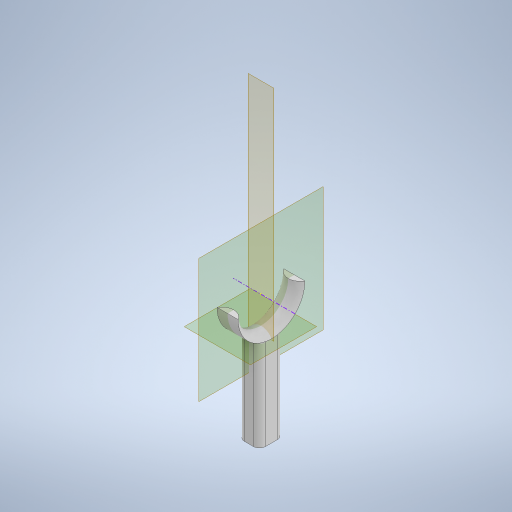
# Autodesk Inventor part: 막대1
Saved by Autodesk Inventor 2023 (Build 270158000, 158)
## iProperties
Created: 2023-04-26
Part Number: 막대1
Material: 일반
Document SubType Name: Modeling
Designer: rlatk
Density: 1 g/cm^3
Appearance: 기본값
Author: rlatk
Autodesk Inventor part; units mm, degrees
ref_plane "YZ Plane" through (0, 0, 0) normal (1, 0, 0) x (0, 1, 0)
ref_plane "XZ Plane" through (0, 0, 0) normal (0, 1, 0) x (-1, 0, 0)
sketch "스케치1" plane through (0, 0, 0) normal (0, 1, 0) x (-1, 0, 0)
  line L0 (0, 0) -> (3.5, 0)
  line L1 (0, 0) -> (-3.5, 0)
  arc A0 (3.5, 0) -> (-3.5, 0) centre (0, -1.9365) ccw
  line L2 (3.5, 0) -> (-3.5, 0)
  dimension "d1" = 3.5
  dimension "d2" = 4
  constraints: 6 end point, 2 point on circle, 1 centre point, 1 collinear, 1 horizontal
  measures "d1" distance of L0.start L0.end
  measures "d2" radius of A0
ref_plane "작업 평면4" through (0, 0, 11.1) normal (0, 0, 1) x (1, 0, 0)
sketch "스케치8" plane through (0, 0, 11.1) normal (0, 0, 1) x (1, 0, 0)
  point P0 (0, 0)
sketch "스케치9" plane through (0, 0, 11.1) normal (0, 0, 1) x (1, 0, 0)
  line L0 (11.2042, 0) -> (-9.3223, 0)
  point P0 (0, 0)
  constraints: 2 end point, 1 horizontal
revolve "회전2" add sketch "스케치1" angle 180 about axis through (11.2042, 0, 11.1) along (-1, 0, 0)
ref_plane "작업 평면5" through (-3.5, -11.1, 11.1) normal (0, -1, 0) x (1, 0, 0)
sketch "스케치10" plane through (-3.5, -11.1, 11.1) normal (0, -1, 0) x (1, 0, 0)
  line L0 (7, 11.1) -> (7, -11.1) projected
  line L1 (7, 0) -> (7, -4)
  line L2 (7, -4) -> (0, -4)
  line L3 (0, 11.1) -> (0, -11.1) projected
  line L4 (0, -4) -> (0, 0)
  line L5 (7, 0) -> (0, 0)
  line L6 (7, -11.1) -> (7, 11.1)
  line L7 (7, 4) -> (0, 4)
  line L8 (0, -11.1) -> (0, 11.1)
  point P0 (3.5, -11.1)
  point P1 (0, 4)
  dimension "d21" = 4
  constraints: 14 end point, 6 symmetric about line, 4 point on line, 2 midpoint, 2 perpendicular
  measures "d21" distance of L1.start L1.end
extrude "돌출4" add sketch "스케치10" along normal blind 30
ref_plane "작업 평면6" through (0, 0, 11.1) normal (-1, 0, 0) x (0, -1, 0)
sketch "스케치11" plane through (0, 0, 11.1) normal (-1, 0, 0) x (0, -1, 0)
  line L0 (11.1, -4) -> (11.1, 0) projected
  line L1 (11.1, -4) -> (10.3542, -4)
  arc A0 (0, -11.1) -> (11.1, 0) centre (0, 0) ccw projected
  line L2 (11.1, -4) -> (11.1, 0)
  arc A1 (10.3542, -4) -> (11.1, 0) centre (0, 0) ccw
  line L3 (11.1, 0) -> (9.0457, 0)
  line L4 (11.1, 4) -> (11.1, 0)
  line L5 (11.1, 4) -> (10.3542, 4)
  arc A2 (11.1, 0) -> (0, 11.1) centre (0, 0) ccw
  arc A3 (11.1, 0) -> (10.3542, 4) centre (0, 0) ccw
  constraints: 10 end point, 8 point on circle, 3 centre point, 3 symmetric about line, 2 horizontal, 1 collinear, 1 concentric, 1 tangent, 2 other
extrude "돌출5" add sketch "스케치11" along normal blind 3.5 and the other way blind 3.5
fillet "모깎기1" radius 2 4 edges at (-3.5, -25.7271, 15.1) (-3.5, -25.7271, 7.1) (3.5, -25.7271, 7.1) (3.5, -25.7271, 15.1)
